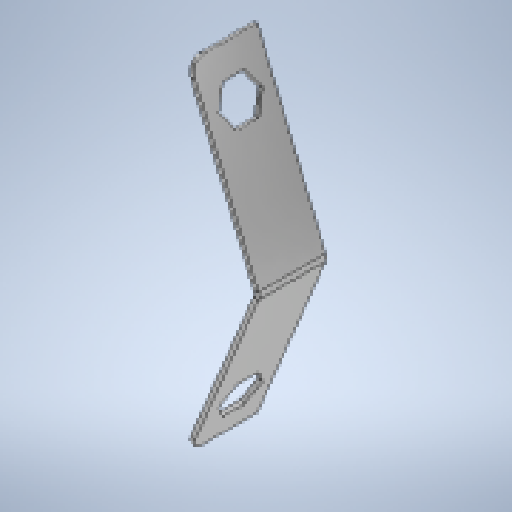
# Autodesk Inventor part: DMF 01 14 Барабан Лист прав брт v2.1
Saved by Autodesk Inventor 2026.2 (Build 302298010, 298A)
## iProperties
Created: 2024-04-28
Part Number: DMF 01 14 Барабан Лист прав брт v2.1
Material: Stainless Steel AISI 304
Document SubType Name: Sheet Metal
Designer: pokla
Density: 8 g/cm^3
Appearance: Chrome - Satin
Sheet Metal Rule: Default
Flat Pattern Width: 16.2262 cm
Flat Pattern Length: 3 cm
Flat Pattern Area: 48.6786 cm^2
Sheet Metal Width: 162,262 mm
Sheet Metal Length: 30,000 mm
Sheet Metal Area: 4867,858 mm^2
Stock Number: Барабан_Лист_Правый_Борт
d174: 145,000 mm
d175: 50,000 mm
Author: pokla
Autodesk Inventor part; units mm, degrees
ref_plane "YZ Plane" through (0, 0, 0) normal (1, 0, 0) x (0, 1, 0)
ref_plane "XZ Plane" through (0, 0, 0) normal (0, 1, 0) x (-1, 0, 0)
ref_plane "XY Plane" through (0, 0, 0) normal (0, 0, 1) x (1, 0, 0)
sketch "Sketch2" plane through (0, 0, 0) normal (0, 0, 1) x (1, 0, 0)
  line L0 (0, 275.468815) -> (194.785867, 194.785867) construction
  line L1 (194.785867, 194.785867) -> (275.468815, 0) construction
  line L2 (275.468815, 0) -> (194.785867, -194.785867) construction
  line L3 (194.785867, -194.785867) -> (0, -275.468815) construction
  line L4 (0, -275.468815) -> (-194.785867, -194.785867) construction
  line L5 (-194.785867, -194.785867) -> (-275.468815, 0) construction
  line L6 (-275.468815, 0) -> (-194.785867, 194.785867) construction
  line L7 (-194.785867, 194.785867) -> (0, 275.468815) construction
  line L8 (244.22009, 75.441096) -> (274.834764, 1.530734)
  line L9 (274.834764, -1.530734) -> (244.22009, -75.441096)
  arc A0 (274.834764, -1.530734) -> (274.834764, 1.530734) centre (271.139246, 0) ccw
  line L10 (275.468815, 0) -> (274.834764, 1.530734) construction
  line L11 (274.834764, 1.530734) -> (276.365498, 2.164784) construction
  line L12 (276.365498, 2.164784) -> (276.999549, 0.634051) construction
  line L13 (276.999549, 0.634051) -> (275.468815, 0) construction
  line L14 (1.530734, 274.834764) -> (0, 275.468815) construction
  line L15 (0, 275.468815) -> (0.634051, 276.999549) construction
  line L16 (0.634051, 276.999549) -> (2.164784, 276.365498) construction
  line L17 (2.164784, 276.365498) -> (1.530734, 274.834764) construction
  point P0 (0, 0)
  point P1 (0, 0)
  dimension "d56" = 509
  dimension "d58" = 4
  dimension "d177" = 80
  measures "d56" distance between parallel lines of L6 L2
  measures "d58" radius of A0
  measures "d177" distance of L8.start L8.end
contour flange "Contour Flange2" sketch "Sketch2" thickness 2 bend radius 2 width 30 along (0, 0, 1) mid plane no both sides no wall seen from (259.527427, 38.485915, 0) lies toward (-0.9238795, -0.3826834, 0) curves L8 A0 L9
bend "Bend2"
corner "Corner2"
sketch "Sketch14" plane through (274.834764, 1.530734, 30) normal (0.9238795, 0.3826834, 0) x (0, 0, -1)
  line L0 (30, 0) -> (0, 0) construction
  line L1 (30, 80) -> (30, 0) construction
  line L2 (0, 80) -> (30, 80)
  line L3 (0, 0) -> (0, 80) construction
  line L4 (24.699485, 60) -> (19.849742, 51.6)
  line L5 (19.849742, 51.6) -> (10.150258, 51.6)
  line L6 (10.150258, 51.6) -> (5.300515, 60)
  line L7 (5.300515, 60) -> (10.150258, 68.4)
  line L8 (10.150258, 68.4) -> (19.849742, 68.4)
  line L9 (19.849742, 68.4) -> (24.699485, 60)
  point P0 (30, 103.760497)
  point P1 (15, 60)
  dimension "d178" = 60
  dimension "d179" = 15
  dimension "d180" = 16.8
  constraints: 12 end point, 1 horizontal, 13 other
  measures "d178" distance from line of L0 point (15, 60)
  measures "d179" distance from line of point (15, 60) L1
  measures "d180" distance between parallel lines of L7 L4
extrude "Cut3" cut sketch "Sketch14" against normal blind 2
mirror "Mirror1" about plane through (0, 0, 0) normal (0, 1, 0) of "Cut3"
fillet "Corner Round1" radius 6 2 edges at (243.2962, 75.0584, 30) (243.2962, -75.0584, 30)
equation "\"d58\" = BendRadius + Thickness"
equation "\"d25\" = Thickness"
equation "\"d26\" = BendReliefWidth"
equation "\"d27\" = BendReliefDepth"
equation "\"d28\" = MinimumRemnant"
equation "\"d29\" = TransitionRadius"
equation "\"d31\" = BendRadius"
equation "\"d33\" = CornerReliefSize"
equation "\"d34\" = GapSize"
equation "\"d35\" = JacobiRadiusSize"
equation "\"GapSize\" = Thickness"
equation "\"BendRadius\" = Thickness"
equation "\"MinimumRemnant\" = 2 * Thickness"
equation "\"BendReliefDepth\" = 0.5 * Thickness"
equation "\"BendReliefWidth\" = Thickness"
equation "\"CornerReliefSize\" = 4 * Thickness"
equation "\"JacobiRadiusSize\" = BendRadius"
equation "\"TransitionRadius\" = BendRadius"
equation "\"d69\" = Барабан_отступ_развертки"
equation "\"d174\" = 145"
equation "\"Thickness\" = 2"
equation "\"Барабан_отступ_развертки\" = 0.9"
body "Solid2"
